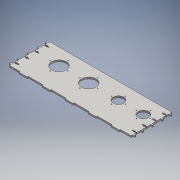
# Autodesk Inventor part: PLANO N°2
Saved by Autodesk Inventor 2016 (Build 200138000, 138)
## iProperties
Created: 2017-09-26
Part Number: PLANO N°2
Material: Genérico
Document SubType Name: Modeling
Designer: Alumno
Density: 1 g/cm^3
Appearance: Valor por defecto
Author: Alumno
Autodesk Inventor part; units mm, degrees
ref_plane "YZ Plane" through (0, 0, 0) normal (1, 0, 0) x (0, 1, 0)
ref_plane "XZ Plane" through (0, 0, 0) normal (0, 1, 0) x (-1, 0, 0)
ref_plane "XY Plane" through (0, 0, 0) normal (0, 0, 1) x (1, 0, 0)
sketch "Boceto1" plane through (0, 0, 0) normal (0, 0, 1) x (1, 0, 0)
  circle A0 centre (-131.4, 15) radius 27
  circle A1 centre (-21.6, 15) radius 27
  circle A2 centre (180, 15) radius 19.5
  circle A3 centre (88.2, 15) radius 19.5
  line L0 (-210, -20.1167) -> (-216, -20.1167)
  line L1 (-216, -20.1167) -> (-216, -21.4167)
  line L2 (-216, -21.4167) -> (-218.8, -21.4167)
  line L3 (-218.8, -21.4167) -> (-218.8, -20.1167)
  line L4 (-218.8, -20.1167) -> (-225, -20.1167)
  line L5 (-225, -20.1167) -> (-225, -34.3833)
  line L6 (-225, -34.3833) -> (-231, -34.3833)
  line L7 (-231, -34.3833) -> (-231, -39.3833)
  line L8 (-225, -39.3833) -> (-231, -39.3833)
  line L9 (-225, -39.3833) -> (-225, -53.65)
  line L10 (-225, -53.65) -> (-218.8, -53.65)
  line L11 (-218.8, -53.65) -> (-218.8, -52.35)
  line L12 (-218.8, -52.35) -> (-216, -52.35)
  line L13 (-216, -52.35) -> (-216, -53.65)
  line L14 (-216, -53.65) -> (-210, -53.65)
  line L15 (-210, -53.65) -> (-210, -57)
  line L16 (-210, -57) -> (-216, -57)
  line L17 (-216, -57) -> (-216, -58.3)
  line L18 (-216, -58.3) -> (-218.8, -58.3)
  line L19 (-218.8, -58.3) -> (-218.8, -57)
  line L20 (-218.8, -57) -> (-225, -57)
  line L21 (-225, -57) -> (-225, -63.5)
  line L22 (-225, -68.5) -> (-225, -75)
  line L23 (-225, -75) -> (-185, -75)
  line L24 (-185, -75) -> (-185, -79)
  line L25 (-185, -79) -> (-155, -79)
  line L26 (-155, -79) -> (-155, -75)
  line L27 (-155, -75) -> (-100, -75)
  line L28 (-100, -75) -> (-100, -79)
  line L29 (-100, -79) -> (-70, -79)
  line L30 (-70, -79) -> (-70, -75)
  line L31 (-70, -75) -> (-15, -75)
  line L32 (-15, -75) -> (-15, -79)
  line L33 (-15, -79) -> (15, -79)
  line L34 (15, -79) -> (15, -75)
  line L35 (15, -75) -> (70, -75)
  line L36 (70, -75) -> (70, -79)
  line L37 (70, -79) -> (100, -79)
  line L38 (100, -79) -> (100, -75)
  line L39 (100, -75) -> (155, -75)
  line L40 (155, -75) -> (155, -79)
  line L41 (155, -79) -> (185, -79)
  line L42 (185, -79) -> (185, -75)
  line L43 (185, -75) -> (225, -75)
  line L44 (225, -75) -> (225, -68.5)
  line L45 (225, -63.5) -> (225, -57)
  line L46 (225, -57) -> (218.8, -57)
  line L47 (218.8, -57) -> (218.8, -58.3)
  line L48 (218.8, -58.3) -> (216, -58.3)
  line L49 (216, -58.3) -> (216, -57)
  line L50 (216, -57) -> (210, -57)
  line L51 (210, -57) -> (210, -53.65)
  line L52 (210, -53.65) -> (216, -53.65)
  line L53 (216, -53.65) -> (216, -52.35)
  line L54 (216, -52.35) -> (218.8, -52.35)
  line L55 (218.8, -52.35) -> (218.8, -53.65)
  line L56 (218.8, -53.65) -> (225, -53.65)
  line L57 (225, -53.65) -> (225, -39.3833)
  line L58 (225, -39.3833) -> (231, -39.3833)
  line L59 (231, -34.3833) -> (231, -39.3833)
  line L60 (225, -34.3833) -> (231, -34.3833)
  line L61 (225, -34.3833) -> (225, -20.1167)
  line L62 (225, -20.1167) -> (218.8, -20.1167)
  line L63 (218.8, -20.1167) -> (218.8, -21.4167)
  line L64 (218.8, -21.4167) -> (216, -21.4167)
  line L65 (216, -21.4167) -> (216, -20.1167)
  line L66 (216, -20.1167) -> (210, -20.1167)
  line L67 (210, -20.1167) -> (210, -16.7667)
  line L68 (210, -16.7667) -> (216, -16.7667)
  line L69 (216, -16.7667) -> (216, -15.4667)
  line L70 (216, -15.4667) -> (218.8, -15.4667)
  line L71 (218.8, -15.4667) -> (218.8, -16.7667)
  line L72 (218.8, -16.7667) -> (225, -16.7667)
  line L73 (225, -16.7667) -> (225, -2.5)
  line L74 (225, -2.5) -> (231, -2.5)
  line L75 (231, 2.5) -> (231, -2.5)
  line L76 (225, 2.5) -> (231, 2.5)
  line L77 (225, 2.5) -> (225, 16.7667)
  line L78 (225, 16.7667) -> (218.8, 16.7667)
  line L79 (218.8, 16.7667) -> (218.8, 15.4667)
  line L80 (218.8, 15.4667) -> (216, 15.4667)
  line L81 (216, 15.4667) -> (216, 16.7667)
  line L82 (216, 16.7667) -> (210, 16.7667)
  line L83 (210, 16.7667) -> (210, 20.1167)
  line L84 (210, 20.1167) -> (216, 20.1167)
  line L85 (216, 20.1167) -> (216, 21.4167)
  line L86 (216, 21.4167) -> (218.8, 21.4167)
  line L87 (218.8, 21.4167) -> (218.8, 20.1167)
  line L88 (218.8, 20.1167) -> (225, 20.1167)
  line L89 (225, 20.1167) -> (225, 34.3833)
  line L90 (225, 34.3833) -> (231, 34.3833)
  line L91 (231, 39.3833) -> (231, 34.3833)
  line L92 (225, 39.3833) -> (231, 39.3833)
  line L93 (225, 39.3833) -> (225, 53.65)
  line L94 (225, 53.65) -> (218.8, 53.65)
  line L95 (218.8, 53.65) -> (218.8, 52.35)
  line L96 (218.8, 52.35) -> (216, 52.35)
  line L97 (216, 52.35) -> (216, 53.65)
  line L98 (216, 53.65) -> (210, 53.65)
  line L99 (210, 53.65) -> (210, 57)
  line L100 (210, 57) -> (216, 57)
  line L101 (216, 57) -> (216, 58.3)
  line L102 (216, 58.3) -> (218.8, 58.3)
  line L103 (218.8, 58.3) -> (218.8, 57)
  line L104 (218.8, 57) -> (225, 57)
  line L105 (225, 57) -> (225, 63.9297)
  line L106 (225, 63.9297) -> (231, 63.9297)
  line L107 (231, 68.9297) -> (231, 63.9297)
  line L108 (225, 68.9297) -> (231, 68.9297)
  line L109 (225, 68.9297) -> (225, 75)
  line L110 (225, 75) -> (-225, 75)
  line L111 (-225, 75) -> (-225, 68.9297)
  line L112 (-225, 68.9297) -> (-231, 68.9297)
  line L113 (-231, 68.9297) -> (-231, 63.9297)
  line L114 (-225, 63.9297) -> (-231, 63.9297)
  line L115 (-225, 63.9297) -> (-225, 57)
  line L116 (-225, 57) -> (-218.8, 57)
  line L117 (-218.8, 57) -> (-218.8, 58.3)
  line L118 (-218.8, 58.3) -> (-216, 58.3)
  line L119 (-216, 58.3) -> (-216, 57)
  line L120 (-216, 57) -> (-210, 57)
  line L121 (-210, 57) -> (-210, 53.65)
  line L122 (-210, 53.65) -> (-216, 53.65)
  line L123 (-216, 53.65) -> (-216, 52.35)
  line L124 (-216, 52.35) -> (-218.8, 52.35)
  line L125 (-218.8, 52.35) -> (-218.8, 53.65)
  line L126 (-218.8, 53.65) -> (-225, 53.65)
  line L127 (-225, 53.65) -> (-225, 39.3833)
  line L128 (-225, 39.3833) -> (-231, 39.3833)
  line L129 (-231, 39.3833) -> (-231, 34.3833)
  line L130 (-225, 34.3833) -> (-231, 34.3833)
  line L131 (-225, 34.3833) -> (-225, 20.1167)
  line L132 (-225, 20.1167) -> (-218.8, 20.1167)
  line L133 (-218.8, 20.1167) -> (-218.8, 21.4167)
  line L134 (-218.8, 21.4167) -> (-216, 21.4167)
  line L135 (-216, 21.4167) -> (-216, 20.1167)
  line L136 (-216, 20.1167) -> (-210, 20.1167)
  line L137 (-210, 20.1167) -> (-210, 16.7667)
  line L138 (-210, 16.7667) -> (-216, 16.7667)
  line L139 (-216, 16.7667) -> (-216, 15.4667)
  line L140 (-216, 15.4667) -> (-218.8, 15.4667)
  line L141 (-218.8, 15.4667) -> (-218.8, 16.7667)
  line L142 (-218.8, 16.7667) -> (-225, 16.7667)
  line L143 (-225, 16.7667) -> (-225, 2.5)
  line L144 (-225, 2.5) -> (-231, 2.5)
  line L145 (-231, 2.5) -> (-231, -2.5)
  line L146 (-225, -2.5) -> (-231, -2.5)
  line L147 (-225, -2.5) -> (-225, -16.7667)
  line L148 (-225, -16.7667) -> (-218.8, -16.7667)
  line L149 (-218.8, -16.7667) -> (-218.8, -15.4667)
  line L150 (-218.8, -15.4667) -> (-216, -15.4667)
  line L151 (-216, -15.4667) -> (-216, -16.7667)
  line L152 (-216, -16.7667) -> (-210, -16.7667)
  line L153 (-210, -16.7667) -> (-210, -20.1167)
  line L154 (-225, -68.5) -> (-231, -68.5)
  line L155 (-231, -68.5) -> (-231, -63.5)
  line L156 (-231, -63.5) -> (-225, -63.5)
  line L157 (225, -63.5) -> (231, -63.5)
  line L158 (231, -63.5) -> (231, -68.5)
  line L159 (231, -68.5) -> (225, -68.5)
  point P0 (0, 0)
  point P1 (0, 0)
  dimension "d2" = 91.8
  dimension "d3" = 450
  dimension "d4" = 150
  dimension "d5" = 45
  dimension "d6" = 109.8
  dimension "d7" = 109.8
  dimension "d8" = 60
  dimension "d11" = 39
  dimension "d12" = 60
  dimension "d13" = 39
  dimension "d14" = 60
  dimension "d15" = 54
  dimension "d16" = 60
  dimension "d17" = 54
  dimension "d48" = 6
  dimension "d51" = 6
  dimension "d52" = 5
  constraints: 320 end point, 4 centre point, 4 perpendicular, 2 horizontal
  measures "d2" distance of A3.centre A2.centre
  measures "d3" distance of L109.end L110.end
  measures "d4" distance between parallel lines of L43 L110
  measures "d5" distance from line of A2.centre L89
  measures "d6" distance of A3.centre A1.centre
  measures "d7" distance of A1.centre A0.centre
  measures "d8" distance from line of L110 A2.centre
  measures "d11" diameter of A2
  measures "d12" distance from line of A3.centre L110
  measures "d13" diameter of A3
  measures "d14" distance from line of A1.centre L110
  measures "d15" diameter of A1
  measures "d16" distance from line of A0.centre L110
  measures "d17" diameter of A0
  measures "d48" distance of L22.start L154.end
  measures "d51" distance of L45.start L157.end
  measures "d52" distance of L157.end L158.end
extrude "Extrusión1" add sketch "Boceto1" along normal blind 6
sketch "Boceto2" plane through (0, 0, 6) normal (0, 0, 1) x (1, 0, 0)
  circle A0 centre (-21.6, 15) radius 27 projected
  circle A1 centre (-131.4, 15) radius 27 projected
  circle A2 centre (88.2, 15) radius 19.5 projected
  circle A3 centre (180, 15) radius 19.5 projected
  line L0 (-210, 57) -> (-210, 53.65) projected
  line L1 (-210, 53.65) -> (-216, 53.65) projected
  line L2 (-216, 53.65) -> (-216, 52.35) projected
  line L3 (-216, 52.35) -> (-218.8, 52.35) projected
  line L4 (-218.8, 52.35) -> (-218.8, 53.65) projected
  line L5 (-218.8, 53.65) -> (-225, 53.65) projected
  line L6 (-225, 53.65) -> (-225, 39.3833) projected
  line L7 (-225, 39.3833) -> (-231, 39.3833) projected
  line L8 (-231, 39.3833) -> (-231, 34.3833) projected
  line L9 (-231, 34.3833) -> (-225, 34.3833) projected
  line L10 (-225, 34.3833) -> (-225, 20.1167) projected
  line L11 (-225, 20.1167) -> (-218.8, 20.1167) projected
  line L12 (-218.8, 20.1167) -> (-218.8, 21.4167) projected
  line L13 (-218.8, 21.4167) -> (-216, 21.4167) projected
  line L14 (-216, 21.4167) -> (-216, 20.1167) projected
  line L15 (-216, 20.1167) -> (-210, 20.1167) projected
  line L16 (-210, 20.1167) -> (-210, 16.7667) projected
  line L17 (-210, 16.7667) -> (-216, 16.7667) projected
  line L18 (-216, 16.7667) -> (-216, 15.4667) projected
  line L19 (-216, 15.4667) -> (-218.8, 15.4667) projected
  line L20 (-218.8, 15.4667) -> (-218.8, 16.7667) projected
  line L21 (-218.8, 16.7667) -> (-225, 16.7667) projected
  line L22 (-225, 16.7667) -> (-225, 2.5) projected
  line L23 (-225, 2.5) -> (-231, 2.5) projected
  line L24 (-231, 2.5) -> (-231, -2.5) projected
  line L25 (-231, -2.5) -> (-225, -2.5) projected
  line L26 (-225, -2.5) -> (-225, -16.7667) projected
  line L27 (-225, -16.7667) -> (-218.8, -16.7667) projected
  line L28 (-218.8, -16.7667) -> (-218.8, -15.4667) projected
  line L29 (-218.8, -15.4667) -> (-216, -15.4667) projected
  line L30 (-216, -15.4667) -> (-216, -16.7667) projected
  line L31 (-216, -16.7667) -> (-210, -16.7667) projected
  line L32 (-210, -16.7667) -> (-210, -20.1167) projected
  line L33 (-210, -20.1167) -> (-216, -20.1167) projected
  line L34 (-216, -20.1167) -> (-216, -21.4167) projected
  line L35 (-216, -21.4167) -> (-218.8, -21.4167) projected
  line L36 (-218.8, -21.4167) -> (-218.8, -20.1167) projected
  line L37 (-218.8, -20.1167) -> (-225, -20.1167) projected
  line L38 (-225, -20.1167) -> (-225, -34.3833) projected
  line L39 (-225, -34.3833) -> (-231, -34.3833) projected
  line L40 (-231, -34.3833) -> (-231, -39.3833) projected
  line L41 (-231, -39.3833) -> (-225, -39.3833) projected
  line L42 (-225, -39.3833) -> (-225, -53.65) projected
  line L43 (-225, -53.65) -> (-218.8, -53.65) projected
  line L44 (-218.8, -53.65) -> (-218.8, -52.35) projected
  line L45 (-218.8, -52.35) -> (-216, -52.35) projected
  line L46 (-216, -52.35) -> (-216, -53.65) projected
  line L47 (-216, -53.65) -> (-210, -53.65) projected
  line L48 (-210, -53.65) -> (-210, -57) projected
  line L49 (-210, -57) -> (-216, -57) projected
  line L50 (-216, -57) -> (-216, -58.3) projected
  line L51 (-216, -58.3) -> (-218.8, -58.3) projected
  line L52 (-218.8, -58.3) -> (-218.8, -57) projected
  line L53 (-218.8, -57) -> (-225, -57) projected
  line L54 (-225, -57) -> (-225, -63.5) projected
  line L55 (-225, -68.5) -> (-225, -75) projected
  line L56 (-225, -75) -> (-185, -75) projected
  line L57 (-185, -75) -> (-185, -79) projected
  line L58 (-185, -79) -> (-155, -79) projected
  line L59 (-155, -79) -> (-155, -75) projected
  line L60 (-155, -75) -> (-100, -75) projected
  line L61 (-100, -75) -> (-100, -79) projected
  line L62 (-100, -79) -> (-70, -79) projected
  line L63 (-70, -79) -> (-70, -75) projected
  line L64 (-70, -75) -> (-15, -75) projected
  line L65 (-15, -75) -> (-15, -79) projected
  line L66 (-15, -79) -> (15, -79) projected
  line L67 (15, -79) -> (15, -75) projected
  line L68 (15, -75) -> (70, -75) projected
  line L69 (70, -75) -> (70, -79) projected
  line L70 (70, -79) -> (100, -79) projected
  line L71 (100, -79) -> (100, -75) projected
  line L72 (100, -75) -> (155, -75) projected
  line L73 (155, -75) -> (155, -79) projected
  line L74 (155, -79) -> (185, -79) projected
  line L75 (185, -79) -> (185, -75) projected
  line L76 (185, -75) -> (225, -75) projected
  line L77 (225, -75) -> (225, -68.5) projected
  line L78 (225, -63.5) -> (225, -57) projected
  line L79 (225, -57) -> (218.8, -57) projected
  line L80 (218.8, -57) -> (218.8, -58.3) projected
  line L81 (218.8, -58.3) -> (216, -58.3) projected
  line L82 (216, -58.3) -> (216, -57) projected
  line L83 (216, -57) -> (210, -57) projected
  line L84 (210, -57) -> (210, -53.65) projected
  line L85 (210, -53.65) -> (216, -53.65) projected
  line L86 (216, -53.65) -> (216, -52.35) projected
  line L87 (216, -52.35) -> (218.8, -52.35) projected
  line L88 (218.8, -52.35) -> (218.8, -53.65) projected
  line L89 (218.8, -53.65) -> (225, -53.65) projected
  line L90 (225, -53.65) -> (225, -39.3833) projected
  line L91 (225, -39.3833) -> (231, -39.3833) projected
  line L92 (231, -39.3833) -> (231, -34.3833) projected
  line L93 (231, -34.3833) -> (225, -34.3833) projected
  line L94 (225, -34.3833) -> (225, -20.1167) projected
  line L95 (225, -20.1167) -> (218.8, -20.1167) projected
  line L96 (218.8, -20.1167) -> (218.8, -21.4167) projected
  line L97 (218.8, -21.4167) -> (216, -21.4167) projected
  line L98 (216, -21.4167) -> (216, -20.1167) projected
  line L99 (216, -20.1167) -> (210, -20.1167) projected
  line L100 (210, -20.1167) -> (210, -16.7667) projected
  line L101 (210, -16.7667) -> (216, -16.7667) projected
  line L102 (216, -16.7667) -> (216, -15.4667) projected
  line L103 (216, -15.4667) -> (218.8, -15.4667) projected
  line L104 (218.8, -15.4667) -> (218.8, -16.7667) projected
  line L105 (218.8, -16.7667) -> (225, -16.7667) projected
  line L106 (225, -16.7667) -> (225, -2.5) projected
  line L107 (225, -2.5) -> (231, -2.5) projected
  line L108 (231, -2.5) -> (231, 2.5) projected
  line L109 (231, 2.5) -> (225, 2.5) projected
  line L110 (225, 2.5) -> (225, 16.7667) projected
  line L111 (225, 16.7667) -> (218.8, 16.7667) projected
  line L112 (218.8, 16.7667) -> (218.8, 15.4667) projected
  line L113 (218.8, 15.4667) -> (216, 15.4667) projected
  line L114 (216, 15.4667) -> (216, 16.7667) projected
  line L115 (216, 16.7667) -> (210, 16.7667) projected
  line L116 (210, 16.7667) -> (210, 20.1167) projected
  line L117 (210, 20.1167) -> (216, 20.1167) projected
  line L118 (216, 20.1167) -> (216, 21.4167) projected
  line L119 (216, 21.4167) -> (218.8, 21.4167) projected
  line L120 (218.8, 21.4167) -> (218.8, 20.1167) projected
  line L121 (218.8, 20.1167) -> (225, 20.1167) projected
  line L122 (225, 20.1167) -> (225, 34.3833) projected
  line L123 (225, 34.3833) -> (231, 34.3833) projected
  line L124 (231, 34.3833) -> (231, 39.3833) projected
  line L125 (231, 39.3833) -> (225, 39.3833) projected
  line L126 (225, 39.3833) -> (225, 53.65) projected
  line L127 (225, 53.65) -> (218.8, 53.65) projected
  line L128 (218.8, 53.65) -> (218.8, 52.35) projected
  line L129 (218.8, 52.35) -> (216, 52.35) projected
  line L130 (216, 52.35) -> (216, 53.65) projected
  line L131 (216, 53.65) -> (210, 53.65) projected
  line L132 (210, 53.65) -> (210, 57) projected
  line L133 (210, 57) -> (216, 57) projected
  line L134 (216, 57) -> (216, 58.3) projected
  line L135 (216, 58.3) -> (218.8, 58.3) projected
  line L136 (218.8, 58.3) -> (218.8, 57) projected
  line L137 (218.8, 57) -> (225, 57) projected
  line L138 (225, 57) -> (225, 63.9297) projected
  line L139 (225, 63.9297) -> (231, 63.9297) projected
  line L140 (231, 63.9297) -> (231, 68.9297) projected
  line L141 (231, 68.9297) -> (225, 68.9297) projected
  line L142 (225, 68.9297) -> (225, 75) projected
  line L143 (225, 75) -> (-225, 75) projected
  line L144 (-225, 75) -> (-225, 68.9297) projected
  line L145 (-225, 68.9297) -> (-231, 68.9297) projected
  line L146 (-231, 68.9297) -> (-231, 63.9297) projected
  line L147 (-231, 63.9297) -> (-225, 63.9297) projected
  line L148 (-225, 63.9297) -> (-225, 57) projected
  line L149 (-225, 57) -> (-218.8, 57) projected
  line L150 (-218.8, 57) -> (-218.8, 58.3) projected
  line L151 (-218.8, 58.3) -> (-216, 58.3) projected
  line L152 (-216, 58.3) -> (-216, 57) projected
  line L153 (-216, 57) -> (-210, 57) projected
  circle A4 centre (-131.4, 48) radius 1.5
  circle A5 centre (-21.6, 48) radius 1.5
  circle A6 centre (-164.4, 15) radius 1.5
  circle A7 centre (-131.4, -18) radius 1.5
  circle A8 centre (-98.4, 15) radius 1.5
  circle A9 centre (-54.6, 15) radius 1.5
  circle A10 centre (-21.6, -18) radius 1.5
  circle A11 centre (11.4, 15) radius 1.5
  line L154 (-225, -63.5) -> (-231, -63.5) projected
  line L155 (-231, -63.5) -> (-231, -68.5) projected
  line L156 (-231, -68.5) -> (-225, -68.5) projected
  line L157 (225, -68.5) -> (231, -68.5) projected
  line L158 (231, -68.5) -> (231, -63.5) projected
  line L159 (231, -63.5) -> (225, -63.5) projected
  point P0 (0, 0)
  dimension "d19" = 3
  dimension "d20" = 33
  dimension "d21" = 3
  dimension "d22" = 33
  dimension "d25" = 360
  dimension "d29" = 360
  constraints: 8 centre point, 18 other
  measures "d19" diameter of A4
  measures "d20" distance of A1.centre A4.centre
  measures "d21" diameter of A5
  measures "d22" distance of A0.centre A5.centre
extrude "Extrusión2" cut sketch "Boceto2" against normal blind 10 contours A4 | A5 | A6 | A7 | A8 | A9 | A10 | A11
sketch "Boceto3" plane through (0, 0, 6) normal (0, 0, 1) x (1, 0, 0)
  circle A0 centre (-21.6, -18) radius 1.5 projected
  circle A1 centre (-98.4, 15) radius 1.5 projected
  circle A2 centre (-164.4, 15) radius 1.5 projected
  circle A3 centre (-131.4, 48) radius 1.5 projected
  circle A4 centre (-21.6, 48) radius 1.5 projected
  circle A5 centre (-131.4, -18) radius 1.5 projected
  circle A6 centre (-54.6, 15) radius 1.5 projected
  circle A7 centre (11.4, 15) radius 1.5 projected
  circle A8 centre (-21.6, 15) radius 27 projected
  circle A9 centre (-131.4, 15) radius 27 projected
  circle A10 centre (88.2, 15) radius 19.5 projected
  circle A11 centre (180, 15) radius 19.5 projected
  line L0 (-210, 57) -> (-210, 53.65) projected
  line L1 (-210, 53.65) -> (-216, 53.65) projected
  line L2 (-216, 53.65) -> (-216, 52.35) projected
  line L3 (-216, 52.35) -> (-218.8, 52.35) projected
  line L4 (-218.8, 52.35) -> (-218.8, 53.65) projected
  line L5 (-218.8, 53.65) -> (-225, 53.65) projected
  line L6 (-225, 53.65) -> (-225, 39.3833) projected
  line L7 (-225, 39.3833) -> (-231, 39.3833) projected
  line L8 (-231, 39.3833) -> (-231, 34.3833) projected
  line L9 (-231, 34.3833) -> (-225, 34.3833) projected
  line L10 (-225, 34.3833) -> (-225, 20.1167) projected
  line L11 (-225, 20.1167) -> (-218.8, 20.1167) projected
  line L12 (-218.8, 20.1167) -> (-218.8, 21.4167) projected
  line L13 (-218.8, 21.4167) -> (-216, 21.4167) projected
  line L14 (-216, 21.4167) -> (-216, 20.1167) projected
  line L15 (-216, 20.1167) -> (-210, 20.1167) projected
  line L16 (-210, 20.1167) -> (-210, 16.7667) projected
  line L17 (-210, 16.7667) -> (-216, 16.7667) projected
  line L18 (-216, 16.7667) -> (-216, 15.4667) projected
  line L19 (-216, 15.4667) -> (-218.8, 15.4667) projected
  line L20 (-218.8, 15.4667) -> (-218.8, 16.7667) projected
  line L21 (-218.8, 16.7667) -> (-225, 16.7667) projected
  line L22 (-225, 16.7667) -> (-225, 2.5) projected
  line L23 (-225, 2.5) -> (-231, 2.5) projected
  line L24 (-231, 2.5) -> (-231, -2.5) projected
  line L25 (-231, -2.5) -> (-225, -2.5) projected
  line L26 (-225, -2.5) -> (-225, -16.7667) projected
  line L27 (-225, -16.7667) -> (-218.8, -16.7667) projected
  line L28 (-218.8, -16.7667) -> (-218.8, -15.4667) projected
  line L29 (-218.8, -15.4667) -> (-216, -15.4667) projected
  line L30 (-216, -15.4667) -> (-216, -16.7667) projected
  line L31 (-216, -16.7667) -> (-210, -16.7667) projected
  line L32 (-210, -16.7667) -> (-210, -20.1167) projected
  line L33 (-210, -20.1167) -> (-216, -20.1167) projected
  line L34 (-216, -20.1167) -> (-216, -21.4167) projected
  line L35 (-216, -21.4167) -> (-218.8, -21.4167) projected
  line L36 (-218.8, -21.4167) -> (-218.8, -20.1167) projected
  line L37 (-218.8, -20.1167) -> (-225, -20.1167) projected
  line L38 (-225, -20.1167) -> (-225, -34.3833) projected
  line L39 (-225, -34.3833) -> (-231, -34.3833) projected
  line L40 (-231, -34.3833) -> (-231, -39.3833) projected
  line L41 (-231, -39.3833) -> (-225, -39.3833) projected
  line L42 (-225, -39.3833) -> (-225, -53.65) projected
  line L43 (-225, -53.65) -> (-218.8, -53.65) projected
  line L44 (-218.8, -53.65) -> (-218.8, -52.35) projected
  line L45 (-218.8, -52.35) -> (-216, -52.35) projected
  line L46 (-216, -52.35) -> (-216, -53.65) projected
  line L47 (-216, -53.65) -> (-210, -53.65) projected
  line L48 (-210, -53.65) -> (-210, -57) projected
  line L49 (-210, -57) -> (-216, -57) projected
  line L50 (-216, -57) -> (-216, -58.3) projected
  line L51 (-216, -58.3) -> (-218.8, -58.3) projected
  line L52 (-218.8, -58.3) -> (-218.8, -57) projected
  line L53 (-218.8, -57) -> (-225, -57) projected
  line L54 (-225, -57) -> (-225, -63.5) projected
  line L55 (-225, -68.5) -> (-225, -75) projected
  line L56 (-225, -75) -> (-185, -75) projected
  line L57 (-185, -75) -> (-185, -79) projected
  line L58 (-185, -79) -> (-155, -79) projected
  line L59 (-155, -79) -> (-155, -75) projected
  line L60 (-155, -75) -> (-100, -75) projected
  line L61 (-100, -75) -> (-100, -79) projected
  line L62 (-100, -79) -> (-70, -79) projected
  line L63 (-70, -79) -> (-70, -75) projected
  line L64 (-70, -75) -> (-15, -75) projected
  line L65 (-15, -75) -> (-15, -79) projected
  line L66 (-15, -79) -> (15, -79) projected
  line L67 (15, -79) -> (15, -75) projected
  line L68 (15, -75) -> (70, -75) projected
  line L69 (70, -75) -> (70, -79) projected
  line L70 (70, -79) -> (100, -79) projected
  line L71 (100, -79) -> (100, -75) projected
  line L72 (100, -75) -> (155, -75) projected
  line L73 (155, -75) -> (155, -79) projected
  line L74 (155, -79) -> (185, -79) projected
  line L75 (185, -79) -> (185, -75) projected
  line L76 (185, -75) -> (225, -75) projected
  line L77 (225, -75) -> (225, -68.5) projected
  line L78 (225, -63.5) -> (225, -57) projected
  line L79 (225, -57) -> (218.8, -57) projected
  line L80 (218.8, -57) -> (218.8, -58.3) projected
  line L81 (218.8, -58.3) -> (216, -58.3) projected
  line L82 (216, -58.3) -> (216, -57) projected
  line L83 (216, -57) -> (210, -57) projected
  line L84 (210, -57) -> (210, -53.65) projected
  line L85 (210, -53.65) -> (216, -53.65) projected
  line L86 (216, -53.65) -> (216, -52.35) projected
  line L87 (216, -52.35) -> (218.8, -52.35) projected
  line L88 (218.8, -52.35) -> (218.8, -53.65) projected
  line L89 (218.8, -53.65) -> (225, -53.65) projected
  line L90 (225, -53.65) -> (225, -39.3833) projected
  line L91 (225, -39.3833) -> (231, -39.3833) projected
  line L92 (231, -39.3833) -> (231, -34.3833) projected
  line L93 (231, -34.3833) -> (225, -34.3833) projected
  line L94 (225, -34.3833) -> (225, -20.1167) projected
  line L95 (225, -20.1167) -> (218.8, -20.1167) projected
  line L96 (218.8, -20.1167) -> (218.8, -21.4167) projected
  line L97 (218.8, -21.4167) -> (216, -21.4167) projected
  line L98 (216, -21.4167) -> (216, -20.1167) projected
  line L99 (216, -20.1167) -> (210, -20.1167) projected
  line L100 (210, -20.1167) -> (210, -16.7667) projected
  line L101 (210, -16.7667) -> (216, -16.7667) projected
  line L102 (216, -16.7667) -> (216, -15.4667) projected
  line L103 (216, -15.4667) -> (218.8, -15.4667) projected
  line L104 (218.8, -15.4667) -> (218.8, -16.7667) projected
  line L105 (218.8, -16.7667) -> (225, -16.7667) projected
  line L106 (225, -16.7667) -> (225, -2.5) projected
  line L107 (225, -2.5) -> (231, -2.5) projected
  line L108 (231, -2.5) -> (231, 2.5) projected
  line L109 (231, 2.5) -> (225, 2.5) projected
  line L110 (225, 2.5) -> (225, 16.7667) projected
  line L111 (225, 16.7667) -> (218.8, 16.7667) projected
  line L112 (218.8, 16.7667) -> (218.8, 15.4667) projected
  line L113 (218.8, 15.4667) -> (216, 15.4667) projected
  line L114 (216, 15.4667) -> (216, 16.7667) projected
  line L115 (216, 16.7667) -> (210, 16.7667) projected
  line L116 (210, 16.7667) -> (210, 20.1167) projected
  line L117 (210, 20.1167) -> (216, 20.1167) projected
  line L118 (216, 20.1167) -> (216, 21.4167) projected
  line L119 (216, 21.4167) -> (218.8, 21.4167) projected
  line L120 (218.8, 21.4167) -> (218.8, 20.1167) projected
  line L121 (218.8, 20.1167) -> (225, 20.1167) projected
  line L122 (225, 20.1167) -> (225, 34.3833) projected
  line L123 (225, 34.3833) -> (231, 34.3833) projected
  line L124 (231, 34.3833) -> (231, 39.3833) projected
  line L125 (231, 39.3833) -> (225, 39.3833) projected
  line L126 (225, 39.3833) -> (225, 53.65) projected
  line L127 (225, 53.65) -> (218.8, 53.65) projected
  line L128 (218.8, 53.65) -> (218.8, 52.35) projected
  line L129 (218.8, 52.35) -> (216, 52.35) projected
  line L130 (216, 52.35) -> (216, 53.65) projected
  line L131 (216, 53.65) -> (210, 53.65) projected
  line L132 (210, 53.65) -> (210, 57) projected
  line L133 (210, 57) -> (216, 57) projected
  line L134 (216, 57) -> (216, 58.3) projected
  line L135 (216, 58.3) -> (218.8, 58.3) projected
  line L136 (218.8, 58.3) -> (218.8, 57) projected
  line L137 (218.8, 57) -> (225, 57) projected
  line L138 (225, 57) -> (225, 63.9297) projected
  line L139 (225, 63.9297) -> (231, 63.9297) projected
  line L140 (231, 63.9297) -> (231, 68.9297) projected
  line L141 (231, 68.9297) -> (225, 68.9297) projected
  line L142 (225, 68.9297) -> (225, 75) projected
  line L143 (225, 75) -> (-225, 75) projected
  line L144 (-225, 75) -> (-225, 68.9297) projected
  line L145 (-225, 68.9297) -> (-231, 68.9297) projected
  line L146 (-231, 68.9297) -> (-231, 63.9297) projected
  line L147 (-231, 63.9297) -> (-225, 63.9297) projected
  line L148 (-225, 63.9297) -> (-225, 57) projected
  line L149 (-225, 57) -> (-218.8, 57) projected
  line L150 (-218.8, 57) -> (-218.8, 58.3) projected
  line L151 (-218.8, 58.3) -> (-216, 58.3) projected
  line L152 (-216, 58.3) -> (-216, 57) projected
  line L153 (-216, 57) -> (-210, 57) projected
  circle A12 centre (88.2, 40.5) radius 1.5
  circle A13 centre (180, 40.5) radius 1.5
  circle A14 centre (62.7, 15) radius 1.5
  circle A15 centre (88.2, -10.5) radius 1.5
  circle A16 centre (113.7, 15) radius 1.5
  circle A17 centre (154.5, 15) radius 1.5
  circle A18 centre (180, -10.5) radius 1.5
  circle A19 centre (205.5, 15) radius 1.5
  line L154 (-225, -63.5) -> (-231, -63.5) projected
  line L155 (-231, -63.5) -> (-231, -68.5) projected
  line L156 (-231, -68.5) -> (-225, -68.5) projected
  line L157 (225, -68.5) -> (231, -68.5) projected
  line L158 (231, -68.5) -> (231, -63.5) projected
  line L159 (231, -63.5) -> (225, -63.5) projected
  point P0 (0, 0)
  dimension "d33" = 3
  dimension "d34" = 25.5
  dimension "d35" = 3
  dimension "d36" = 25.5
  dimension "d39" = 360
  dimension "d43" = 360
  constraints: 8 centre point, 18 other
  measures "d33" diameter of A12
  measures "d34" distance of A10.centre A12.centre
  measures "d35" diameter of A13
  measures "d36" distance of A11.centre A13.centre
extrude "Extrusión3" cut sketch "Boceto3" against normal blind 10 contours A12 | A13 | A14 | A15 | A16 | A17 | A18 | A19
